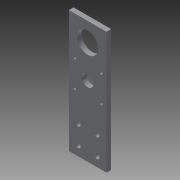
# Autodesk Inventor part: Z-Plate-Gears
Saved by Autodesk Inventor 2013 (Build 170138000, 138)
## iProperties
Created: 2014-01-24
Part Number: Z-Plate-Gears
Material: Generic
Document SubType Name: Modeling
Designer: Jarod
Density: 1 g/cm^3
Author: Jarod
Autodesk Inventor part; units mm, degrees
ref_plane "YZ Plane" through (0, 0, 0) normal (1, 0, 0) x (0, 1, 0)
ref_plane "XZ Plane" through (0, 0, 0) normal (0, 1, 0) x (-1, 0, 0)
ref_plane "XY Plane" through (0, 0, 0) normal (0, 0, 1) x (1, 0, 0)
sketch "Sketch1" plane through (0, 0, 0) normal (0, 0, 1) x (1, 0, 0)
  line L0 (0, 0) -> (50.8, 0)
  line L1 (50.8, 0) -> (50.8, 169.8752)
  line L2 (50.8, 169.8752) -> (0, 169.8752)
  line L3 (0, 169.8752) -> (0, 0)
  line L4 (25.4, 169.8752) -> (25.4, 144.4752)
  line L5 (25.4, 169.8752) -> (50.8, 169.8752) construction
  circle A0 centre (25.4, 144.4752) radius 14.2875
  line L6 (25.4, 144.4752) -> (43.3605, 162.4357)
  line L7 (25.4, 144.4752) -> (50.8, 144.4752) construction
  line L8 (7.4395, 126.5147) -> (43.3605, 126.5147)
  line L9 (43.3605, 162.4357) -> (7.4395, 162.4357)
  line L10 (7.4395, 162.4357) -> (7.4395, 126.5147)
  circle A1 centre (7.4395, 162.4357) radius 2.032
  circle A2 centre (7.4395, 126.5147) radius 2.032
  circle A3 centre (43.3605, 162.4357) radius 2.032
  circle A4 centre (43.3605, 126.5147) radius 2.032
  line L11 (0, 0) -> (50.8, 0)
  line L12 (50.8, 0) -> (50.8, 38.1)
  line L13 (0, 38.1) -> (0, 0)
  line L14 (25.4, 38.1) -> (12.7, 38.1)
  line L15 (25.4, 38.1) -> (38.1, 38.1) construction
  line L16 (12.7, 38.1) -> (38.1, 38.1)
  circle A5 centre (12.7, 38.1) radius 3.175
  circle A6 centre (38.1, 38.1) radius 3.175
  dimension "d0" = 50.8
  dimension "d1" = 169.8752
  dimension "d2" = 25.4
  dimension "d3" = 90
  dimension "d4" = 28.575
  dimension "d5" = 25.4
  dimension "d6" = 45
  dimension "d7" = 50.8
  dimension "d9" = 4.064
  dimension "d10" = 4.064
  dimension "d11" = 4.064
  dimension "d12" = 4.064
  dimension "d13" = 50.8
  dimension "d14" = 38.1
  dimension "d15" = 12.7
  dimension "d16" = 180
  dimension "d17" = 25.4
  dimension "d18" = 0
  dimension "d19" = 6.35
  dimension "d20" = 6.35
  constraints: 34 end point, 7 centre point, 7 coincident, 6 horizontal, 5 parallel, 3 equal length, 2 perpendicular, 1 midpoint
  measures "d0" distance of L2.end L1.end
  measures "d1" distance of L1.end L0.end
  measures "d2" distance of L4.start L4.end
  measures "d3" angle of L4 L5
  measures "d4" diameter of A0
  measures "d5" distance of L6.start L6.end
  measures "d6" angle of L7 L6
  measures "d7" distance of L6.end L8.start
  measures "d9" diameter of A1
  measures "d10" diameter of A2
  measures "d11" diameter of A3
  measures "d12" diameter of A4
  measures "d13" distance of L13.start L12.end
  measures "d14" distance of L12.end L11.end
  measures "d15" distance of L14.start L14.end
  measures "d16" angle of L14 L15
  measures "d17" distance of L14.end L16.end
  measures "d18" distance between parallel lines of L16 L14
  measures "d19" diameter of A5
  measures "d20" diameter of A6
extrude "Extrusion1" add sketch "Sketch1" along normal blind 25.4 contours L9 A3 L6 A0 L4 | L3 L2 L1 L0
sketch "Sketch2" plane through (0, 169.8752, 0) normal (0, 1, 0) x (1, 0, 0)
  line L0 (0, 0) -> (3.175, 0)
  line L1 (3.175, 0) -> (3.175, -3.175)
  line L2 (3.175, -3.175) -> (0, -3.175)
  line L3 (0, -3.175) -> (0, 0)
  line L4 (3.175, -3.175) -> (47.625, -3.175)
  line L5 (47.625, -3.175) -> (47.625, -22.225)
  line L6 (47.625, -22.225) -> (3.175, -22.225)
  line L7 (3.175, -22.225) -> (3.175, -3.175)
  dimension "d23" = 3.175
  dimension "d24" = 3.175
  dimension "d25" = 44.45
  dimension "d26" = 19.05
  constraints: 16 end point, 4 parallel, 2 horizontal, 2 perpendicular
  measures "d23" distance of L1.end L2.end
  measures "d24" distance of L0.end L1.end
  measures "d25" distance of L5.end L6.end
  measures "d26" distance of L4.end L5.end
extrude "Extrusion2" cut sketch "Sketch2" against normal blind 254 contours L4 L5 L6 L7
sketch "Sketch3" plane through (0, 0, 25.4) normal (0, 0, 1) x (1, 0, 0)
  circle A0 centre (12.7, 38.1) radius 3.175 projected
  line L0 (12.7, 38.1) -> (38.1, 38.1)
  line L1 (38.1, 38.1) -> (38.1, 12.7)
  line L2 (38.1, 12.7) -> (12.7, 12.7)
  line L3 (12.7, 12.7) -> (12.7, 38.1)
  circle A1 centre (12.7, 12.7) radius 3.175
  circle A2 centre (38.1, 12.7) radius 3.175
  dimension "d29" = 25.4
  dimension "d30" = 25.4
  dimension "d31" = 6.35
  dimension "d32" = 6.35
  constraints: 8 end point, 2 centre point, 2 coincident, 2 parallel, 1 horizontal, 1 perpendicular
  measures "d29" distance of L1.end L2.end
  measures "d30" distance of L0.end L1.end
  measures "d31" diameter of A1
  measures "d32" diameter of A2
extrude "Extrusion3" cut sketch "Sketch3" against normal blind 25.4 contours A1 L2 L3 | L3 L2 A1 | A2 L2 L1 | L1 L2 A2
sketch "Sketch4" plane through (0, 169.8752, 0) normal (0, 1, 0) x (1, 0, 0)
  line L0 (47.625, -22.225) -> (3.175, -22.225) projected
  line L1 (3.175, -22.225) -> (3.175, -3.175) projected
  line L2 (3.175, -3.175) -> (47.625, -3.175) projected
  line L3 (47.625, -3.175) -> (47.625, -22.225) projected
  line L4 (50.8, 0) -> (50.8, -25.4) projected
  line L5 (0, 0) -> (50.8, 0)
  line L6 (50.8, 0) -> (50.8, -22.225)
  line L7 (50.8, -22.225) -> (0, -22.225)
  line L8 (0, -22.225) -> (0, 0)
  constraints: 8 end point, 2 parallel, 1 horizontal, 1 perpendicular, 1 point on line
extrude "Extrusion4" cut sketch "Sketch4" against normal blind 254 contours L3 L2 L1 L7 L8 L5 L4
sketch "Sketch5" plane through (0, 0, 25.4) normal (0, 0, 1) x (1, 0, 0)
  circle A0 centre (38.1, 12.7) radius 3.175 projected
  circle A1 centre (12.7, 12.7) radius 3.175 projected
  circle A2 centre (25.4, 144.4752) radius 14.2875 projected
  circle A3 centre (38.1, 38.1) radius 3.175 projected
  circle A4 centre (12.7, 38.1) radius 3.175 projected
  circle A5 centre (43.3605, 126.5147) radius 2.032 projected
  circle A6 centre (43.3605, 162.4357) radius 2.032 projected
  circle A7 centre (7.4395, 126.5147) radius 2.032 projected
  circle A8 centre (7.4395, 162.4357) radius 2.032 projected
  line L0 (0, 0) -> (50.8, 0) projected
  line L1 (50.8, 0) -> (50.8, 169.8752) projected
  line L2 (50.8, 169.8752) -> (0, 169.8752) projected
  line L3 (0, 169.8752) -> (0, 0) projected
extrude "Extrusion5" add sketch "Sketch5" along normal blind 3.175
sketch "Sketch6" plane through (0, 0, 28.575) normal (0, 0, 1) x (1, 0, 0)
  circle A0 centre (25.4, 144.4752) radius 14.2875 projected
  circle A1 centre (25.4, 144.4752) radius 9.525
  dimension "d39" = 19.05
  constraints: 1 centre point, 1 coincident
  measures "d39" diameter of A1
extrude "Extrusion6" add sketch "Sketch6" against normal blind 6.35
sketch "Sketch7" plane through (0, 0, 28.575) normal (0, 0, 1) x (1, 0, 0)
  line L0 (50.8, 169.8752) -> (0, 169.8752) projected
  line L1 (0, 169.8752) -> (0, 0) projected
  line L2 (25.4, 169.8752) -> (25.4, 95.25)
  line L3 (25.4, 169.8752) -> (100.0252, 169.8752) construction
  circle A0 centre (25.4, 95.25) radius 7.9375
  dimension "d43" = 74.6252
  dimension "d44" = 90
  dimension "d45" = 15.875
  constraints: 4 end point, 1 centre point, 1 coincident, 1 horizontal, 1 midpoint, 1 parallel, 1 perpendicular
  measures "d43" distance of L2.start L2.end
  measures "d44" angle of L2 L3
  measures "d45" diameter of A0
extrude "Extrusion7" cut sketch "Sketch7" against normal blind 25.4
sketch "Sketch8" plane through (0, 0, 28.575) normal (0, 0, 1) x (1, 0, 0)
  circle A0 centre (25.4, 144.4752) radius 9.525 projected
  circle A1 centre (25.4, 144.4752) radius 14.2875
  dimension "d48" = 28.575
  constraints: 1 centre point, 1 coincident
  measures "d48" diameter of A1
extrude "Extrusion8" cut sketch "Sketch8" against normal blind 25.4
sketch "Sketch9" plane through (0, 0, 28.575) normal (0, 0, 1) x (1, 0, 0)
  circle A0 centre (25.4, 95.25) radius 7.9375 projected
  circle A1 centre (7.4395, 162.4357) radius 2.032 projected
  circle A2 centre (7.4395, 126.5147) radius 2.032 projected
  circle A3 centre (43.3605, 162.4357) radius 2.032 projected
  circle A4 centre (43.3605, 126.5147) radius 2.032 projected
  line L0 (25.4, 95.25) -> (43.3605, 113.2105)
  line L1 (25.4, 95.25) -> (50.8, 95.25) construction
  line L2 (43.3605, 113.2105) -> (7.4395, 77.2895)
  circle A5 centre (7.4395, 113.2105) radius 2.032
  circle A6 centre (43.3605, 113.2105) radius 2.032
  circle A7 centre (43.3605, 77.2895) radius 2.032
  circle A8 centre (7.4395, 77.2895) radius 2.032
  dimension "d51" = 25.4
  dimension "d52" = 45
  dimension "d53" = 50.8
  dimension "d54" = 0
  dimension "d55" = 4.064
  dimension "d56" = 4.064
  dimension "d57" = 4.064
  dimension "d58" = 4.064
  constraints: 6 end point, 4 centre point, 2 coincident, 1 collinear, 1 equal length, 1 horizontal
  measures "d51" distance of L0.start L0.end
  measures "d52" angle of L1 L0
  measures "d53" distance of L0.end L2.end
  measures "d54" distance between parallel lines of L2 L0
  measures "d55" diameter of A5
  measures "d56" diameter of A6
  measures "d57" diameter of A7
  measures "d58" diameter of A8
extrude "Extrusion9" cut sketch "Sketch9" against normal blind 6.35 contours A8 | A6 | A1 | A2 | A3 | A4 | A5 | A7
sketch "Sketch10" plane through (0, 0, 28.575) normal (0, 0, 1) x (1, 0, 0)
  circle A0 centre (7.4395, 162.4357) radius 2.032 projected
  circle A1 centre (7.4395, 126.5147) radius 2.032 projected
  circle A2 centre (43.3605, 162.4357) radius 2.032 projected
  circle A3 centre (43.3605, 126.5147) radius 2.032 projected
extrude "Extrusion10" add sketch "Sketch10" against normal blind 6.35
sketch "Sketch11" plane through (0, 0, 28.575) normal (0, 0, 1) x (1, 0, 0)
  circle A0 centre (25.4, 144.4752) radius 14.2875 projected
  line L0 (0, 169.8752) -> (50.8, 169.8752)
  line L1 (50.8, 169.8752) -> (50.8, 119.0752)
  line L2 (50.8, 119.0752) -> (0, 119.0752)
  line L3 (0, 119.0752) -> (0, 169.8752)
  dimension "d64" = 50.8
  dimension "d65" = 50.8
  constraints: 8 end point, 2 parallel, 1 horizontal, 1 perpendicular
  measures "d64" distance of L1.end L2.end
  measures "d65" distance of L0.end L1.end
extrude "Extrusion11" cut sketch "Sketch11" against normal blind 25.4
sketch "Sketch12" plane through (0, 0, 28.575) normal (0, 0, 1) x (1, 0, 0)
  line L0 (50.8, 0) -> (50.8, 119.0752) projected
  circle A0 centre (25.4, 95.25) radius 7.9375 projected
  line L1 (25.4, 95.25) -> (25.4, 139.7)
  line L2 (25.4, 95.25) -> (69.85, 95.25) construction
  circle A1 centre (25.4, 139.7) radius 14.2875
  line L3 (25.4, 139.7) -> (25.4, 165.1)
  line L4 (25.4, 139.7) -> (50.8, 139.7) construction
  line L5 (25.4, 165.1) -> (0, 165.1)
  line L6 (0, 165.1) -> (50.8, 165.1)
  line L7 (50.8, 165.1) -> (50.8, 119.0752)
  line L8 (50.8, 119.0752) -> (0, 119.0752)
  line L9 (0, 119.0752) -> (0, 165.1)
  dimension "d68" = 44.45
  dimension "d69" = 90
  dimension "d70" = 28.575
  dimension "d71" = 25.4
  dimension "d72" = 90
  dimension "d73" = 25.4
  dimension "d74" = 90
  constraints: 18 end point, 5 perpendicular, 3 horizontal, 3 parallel, 1 centre point, 1 coincident
  measures "d68" distance of L1.start L1.end
  measures "d69" angle of L2 L1
  measures "d70" diameter of A1
  measures "d71" distance of L3.start L3.end
  measures "d72" angle of L4 L3
  measures "d73" distance of L3.end L5.end
  measures "d74" angle of L5 L3
extrude "Extrusion12" add sketch "Sketch12" against normal blind 6.35 contours L8 L9 L5 L3 A1 L1 | L1 A1 L3 L6 L7 L8
body "Solid1"
